Autodesk Fusion 360 part; units mm, degrees
(part 8 of 12)
  line L2696 (39.3845, 201.3731) -> (39.3845, 206.3731)
  line L2697 (39.3845, 206.3731) -> (35.0544, 208.8731)
  line L2698 (45.7146, 208.8731) -> (41.3845, 206.3731)
  line L2699 (41.3845, 206.3731) -> (41.3845, 201.3731)
  line L2700 (41.3845, 201.3731) -> (45.7146, 198.8731)
  line L2701 (45.7146, 198.8731) -> (50.0447, 201.3731)
  line L2702 (50.0447, 201.3731) -> (50.0447, 206.3731)
  line L2703 (50.0447, 206.3731) -> (45.7146, 208.8731)
  line L2704 (56.3749, 208.8731) -> (52.0447, 206.3731)
  line L2705 (52.0447, 206.3731) -> (52.0447, 201.3731)
  line L2706 (52.0447, 201.3731) -> (56.3749, 198.8731)
  line L2707 (56.3749, 198.8731) -> (60.705, 201.3731)
  line L2708 (60.705, 201.3731) -> (60.705, 206.3731)
  line L2709 (60.705, 206.3731) -> (56.3749, 208.8731)
  line L2710 (-151.5001, 218.1051) -> (-155.8302, 215.6051)
  line L2711 (-155.8302, 215.6051) -> (-155.8302, 210.6051)
  line L2712 (-155.8302, 210.6051) -> (-151.5001, 208.1051)
  line L2713 (-151.5001, 208.1051) -> (-147.17, 210.6051)
  line L2714 (-147.17, 210.6051) -> (-147.17, 215.6051)
  line L2715 (-147.17, 215.6051) -> (-151.5001, 218.1051)
  line L2716 (-140.8398, 218.1051) -> (-145.17, 215.6051)
  line L2717 (-145.17, 215.6051) -> (-145.17, 210.6051)
  line L2718 (-145.17, 210.6051) -> (-140.8398, 208.1051)
  line L2719 (-140.8398, 208.1051) -> (-136.5097, 210.6051)
  line L2720 (-136.5097, 210.6051) -> (-136.5097, 215.6051)
  line L2721 (-136.5097, 215.6051) -> (-140.8398, 218.1051)
  line L2722 (-130.1796, 218.1051) -> (-134.5097, 215.6051)
  line L2723 (-134.5097, 215.6051) -> (-134.5097, 210.6051)
  line L2724 (-134.5097, 210.6051) -> (-130.1796, 208.1051)
  line L2725 (-130.1796, 208.1051) -> (-125.8494, 210.6051)
  line L2726 (-125.8494, 210.6051) -> (-125.8494, 215.6051)
  line L2727 (-125.8494, 215.6051) -> (-130.1796, 218.1051)
  line L2728 (-119.5193, 218.1051) -> (-123.8494, 215.6051)
  line L2729 (-123.8494, 215.6051) -> (-123.8494, 210.6051)
  line L2730 (-123.8494, 210.6051) -> (-119.5193, 208.1051)
  line L2731 (-119.5193, 208.1051) -> (-115.1892, 210.6051)
  line L2732 (-115.1892, 210.6051) -> (-115.1892, 215.6051)
  line L2733 (-115.1892, 215.6051) -> (-119.5193, 218.1051)
  line L2734 (-108.8591, 218.1051) -> (-113.1892, 215.6051)
  line L2735 (-113.1892, 215.6051) -> (-113.1892, 210.6051)
  line L2736 (-113.1892, 210.6051) -> (-108.8591, 208.1051)
  line L2737 (-108.8591, 208.1051) -> (-104.5289, 210.6051)
  line L2738 (-104.5289, 210.6051) -> (-104.5289, 215.6051)
  line L2739 (-104.5289, 215.6051) -> (-108.8591, 218.1051)
  line L2740 (-98.1988, 218.1051) -> (-102.5289, 215.6051)
  line L2741 (-102.5289, 215.6051) -> (-102.5289, 210.6051)
  line L2742 (-102.5289, 210.6051) -> (-98.1988, 208.1051)
  line L2743 (-98.1988, 208.1051) -> (-93.8687, 210.6051)
  line L2744 (-93.8687, 210.6051) -> (-93.8687, 215.6051)
  line L2745 (-93.8687, 215.6051) -> (-98.1988, 218.1051)
  line L2746 (-87.5386, 218.1051) -> (-91.8687, 215.6051)
  line L2747 (-91.8687, 215.6051) -> (-91.8687, 210.6051)
  line L2748 (-91.8687, 210.6051) -> (-87.5386, 208.1051)
  line L2749 (-87.5386, 208.1051) -> (-83.2084, 210.6051)
  line L2750 (-83.2084, 210.6051) -> (-83.2084, 215.6051)
  line L2751 (-83.2084, 215.6051) -> (-87.5386, 218.1051)
  line L2752 (-76.8783, 218.1051) -> (-81.2084, 215.6051)
  line L2753 (-81.2084, 215.6051) -> (-81.2084, 210.6051)
  line L2754 (-81.2084, 210.6051) -> (-76.8783, 208.1051)
  line L2755 (-76.8783, 208.1051) -> (-72.5482, 210.6051)
  line L2756 (-72.5482, 210.6051) -> (-72.5482, 215.6051)
  line L2757 (-72.5482, 215.6051) -> (-76.8783, 218.1051)
  line L2758 (-66.218, 218.1051) -> (-70.5482, 215.6051)
  line L2759 (-70.5482, 215.6051) -> (-70.5482, 210.6051)
  line L2760 (-70.5482, 210.6051) -> (-66.218, 208.1051)
  line L2761 (-66.218, 208.1051) -> (-61.8879, 210.6051)
  line L2762 (-61.8879, 210.6051) -> (-61.8879, 215.6051)
  line L2763 (-61.8879, 215.6051) -> (-66.218, 218.1051)
  line L2764 (-55.5578, 218.1051) -> (-59.8879, 215.6051)
  line L2765 (-59.8879, 215.6051) -> (-59.8879, 210.6051)
  line L2766 (-59.8879, 210.6051) -> (-55.5578, 208.1051)
  line L2767 (-55.5578, 208.1051) -> (-51.2277, 210.6051)
  line L2768 (-51.2277, 210.6051) -> (-51.2277, 215.6051)
  line L2769 (-51.2277, 215.6051) -> (-55.5578, 218.1051)
  line L2770 (-44.8975, 218.1051) -> (-49.2277, 215.6051)
  line L2771 (-49.2277, 215.6051) -> (-49.2277, 210.6051)
  line L2772 (-49.2277, 210.6051) -> (-44.8975, 208.1051)
  line L2773 (-44.8975, 208.1051) -> (-40.5674, 210.6051)
  line L2774 (-40.5674, 210.6051) -> (-40.5674, 215.6051)
  line L2775 (-40.5674, 215.6051) -> (-44.8975, 218.1051)
  line L2776 (-34.2373, 218.1051) -> (-38.5674, 215.6051)
  line L2777 (-38.5674, 215.6051) -> (-38.5674, 210.6051)
  line L2778 (-38.5674, 210.6051) -> (-34.2373, 208.1051)
  line L2779 (-34.2373, 208.1051) -> (-29.9072, 210.6051)
  line L2780 (-29.9072, 210.6051) -> (-29.9072, 215.6051)
  line L2781 (-29.9072, 215.6051) -> (-34.2373, 218.1051)
  line L2782 (-23.577, 218.1051) -> (-27.9072, 215.6051)
  line L2783 (-27.9072, 215.6051) -> (-27.9072, 210.6051)
  line L2784 (-27.9072, 210.6051) -> (-23.577, 208.1051)
  line L2785 (-23.577, 208.1051) -> (-19.2469, 210.6051)
  line L2786 (-19.2469, 210.6051) -> (-19.2469, 215.6051)
  line L2787 (-19.2469, 215.6051) -> (-23.577, 218.1051)
  line L2788 (-12.9168, 218.1051) -> (-17.2469, 215.6051)
  line L2789 (-17.2469, 215.6051) -> (-17.2469, 210.6051)
  line L2790 (-17.2469, 210.6051) -> (-12.9168, 208.1051)
  line L2791 (-12.9168, 208.1051) -> (-8.5866, 210.6051)
  line L2792 (-8.5866, 210.6051) -> (-8.5866, 215.6051)
  line L2793 (-8.5866, 215.6051) -> (-12.9168, 218.1051)
  line L2794 (-2.2565, 218.1051) -> (-6.5866, 215.6051)
  line L2795 (-6.5866, 215.6051) -> (-6.5866, 210.6051)
  line L2796 (-6.5866, 210.6051) -> (-2.2565, 208.1051)
  line L2797 (-2.2565, 208.1051) -> (2.0736, 210.6051)
  line L2798 (2.0736, 210.6051) -> (2.0736, 215.6051)
  line L2799 (2.0736, 215.6051) -> (-2.2565, 218.1051)
  line L2800 (8.4037, 218.1051) -> (4.0736, 215.6051)
  line L2801 (4.0736, 215.6051) -> (4.0736, 210.6051)
  line L2802 (4.0736, 210.6051) -> (8.4037, 208.1051)
  line L2803 (8.4037, 208.1051) -> (12.7339, 210.6051)
  line L2804 (12.7339, 210.6051) -> (12.7339, 215.6051)
  line L2805 (12.7339, 215.6051) -> (8.4037, 218.1051)
  line L2806 (19.064, 218.1051) -> (14.7339, 215.6051)
  line L2807 (14.7339, 215.6051) -> (14.7339, 210.6051)
  line L2808 (14.7339, 210.6051) -> (19.064, 208.1051)
  line L2809 (19.064, 208.1051) -> (23.3941, 210.6051)
  line L2810 (23.3941, 210.6051) -> (23.3941, 215.6051)
  line L2811 (23.3941, 215.6051) -> (19.064, 218.1051)
  line L2812 (29.7242, 218.1051) -> (25.3941, 215.6051)
  line L2813 (25.3941, 215.6051) -> (25.3941, 210.6051)
  line L2814 (25.3941, 210.6051) -> (29.7242, 208.1051)
  line L2815 (29.7242, 208.1051) -> (34.0544, 210.6051)
  line L2816 (34.0544, 210.6051) -> (34.0544, 215.6051)
  line L2817 (34.0544, 215.6051) -> (29.7242, 218.1051)
  line L2818 (40.3845, 218.1051) -> (36.0544, 215.6051)
  line L2819 (36.0544, 215.6051) -> (36.0544, 210.6051)
  line L2820 (36.0544, 210.6051) -> (40.3845, 208.1051)
  line L2821 (40.3845, 208.1051) -> (44.7146, 210.6051)
  line L2822 (44.7146, 210.6051) -> (44.7146, 215.6051)
  line L2823 (44.7146, 215.6051) -> (40.3845, 218.1051)
  line L2824 (51.0447, 218.1051) -> (46.7146, 215.6051)
  line L2825 (46.7146, 215.6051) -> (46.7146, 210.6051)
  line L2826 (46.7146, 210.6051) -> (51.0447, 208.1051)
  line L2827 (51.0447, 208.1051) -> (55.3749, 210.6051)
  line L2828 (55.3749, 210.6051) -> (55.3749, 215.6051)
  line L2829 (55.3749, 215.6051) -> (51.0447, 218.1051)
  line L2830 (61.705, 218.1051) -> (57.3749, 215.6051)
  line L2831 (57.3749, 215.6051) -> (57.3749, 210.6051)
  line L2832 (57.3749, 210.6051) -> (61.705, 208.1051)
  line L2833 (61.705, 208.1051) -> (66.0351, 210.6051)
  line L2834 (66.0351, 210.6051) -> (66.0351, 215.6051)
  line L2835 (66.0351, 215.6051) -> (61.705, 218.1051)
  line L2836 (-146.17, 227.3372) -> (-150.5001, 224.8372)
  line L2837 (-150.5001, 224.8372) -> (-150.5001, 219.8372)
  line L2838 (-150.5001, 219.8372) -> (-146.17, 217.3372)
  line L2839 (-146.17, 217.3372) -> (-141.8398, 219.8372)
  line L2840 (-141.8398, 219.8372) -> (-141.8398, 224.8372)
  line L2841 (-141.8398, 224.8372) -> (-146.17, 227.3372)
  line L2842 (-135.5097, 227.3372) -> (-139.8398, 224.8372)
  line L2843 (-139.8398, 224.8372) -> (-139.8398, 219.8372)
  line L2844 (-139.8398, 219.8372) -> (-135.5097, 217.3372)
  line L2845 (-135.5097, 217.3372) -> (-131.1796, 219.8372)
  line L2846 (-131.1796, 219.8372) -> (-131.1796, 224.8372)
  line L2847 (-131.1796, 224.8372) -> (-135.5097, 227.3372)
  line L2848 (-124.8494, 227.3372) -> (-129.1796, 224.8372)
  line L2849 (-129.1796, 224.8372) -> (-129.1796, 219.8372)
  line L2850 (-129.1796, 219.8372) -> (-124.8494, 217.3372)
  line L2851 (-124.8494, 217.3372) -> (-120.5193, 219.8372)
  line L2852 (-120.5193, 219.8372) -> (-120.5193, 224.8372)
  line L2853 (-120.5193, 224.8372) -> (-124.8494, 227.3372)
  line L2854 (-114.1892, 227.3372) -> (-118.5193, 224.8372)
  line L2855 (-118.5193, 224.8372) -> (-118.5193, 219.8372)
  line L2856 (-118.5193, 219.8372) -> (-114.1892, 217.3372)
  line L2857 (-114.1892, 217.3372) -> (-109.8591, 219.8372)
  line L2858 (-109.8591, 219.8372) -> (-109.8591, 224.8372)
  line L2859 (-109.8591, 224.8372) -> (-114.1892, 227.3372)
  line L2860 (-103.5289, 227.3372) -> (-107.8591, 224.8372)
  line L2861 (-107.8591, 224.8372) -> (-107.8591, 219.8372)
  line L2862 (-107.8591, 219.8372) -> (-103.5289, 217.3372)
  line L2863 (-103.5289, 217.3372) -> (-99.1988, 219.8372)
  line L2864 (-99.1988, 219.8372) -> (-99.1988, 224.8372)
  line L2865 (-99.1988, 224.8372) -> (-103.5289, 227.3372)
  line L2866 (-92.8687, 227.3372) -> (-97.1988, 224.8372)
  line L2867 (-97.1988, 224.8372) -> (-97.1988, 219.8372)
  line L2868 (-97.1988, 219.8372) -> (-92.8687, 217.3372)
  line L2869 (-92.8687, 217.3372) -> (-88.5386, 219.8372)
  line L2870 (-88.5386, 219.8372) -> (-88.5386, 224.8372)
  line L2871 (-88.5386, 224.8372) -> (-92.8687, 227.3372)
  line L2872 (-82.2084, 227.3372) -> (-86.5386, 224.8372)
  line L2873 (-86.5386, 224.8372) -> (-86.5386, 219.8372)
  line L2874 (-86.5386, 219.8372) -> (-82.2084, 217.3372)
  line L2875 (-82.2084, 217.3372) -> (-77.8783, 219.8372)
  line L2876 (-77.8783, 219.8372) -> (-77.8783, 224.8372)
  line L2877 (-77.8783, 224.8372) -> (-82.2084, 227.3372)
  line L2878 (-71.5482, 227.3372) -> (-75.8783, 224.8372)
  line L2879 (-75.8783, 224.8372) -> (-75.8783, 219.8372)
  line L2880 (-75.8783, 219.8372) -> (-71.5482, 217.3372)
  line L2881 (-71.5482, 217.3372) -> (-67.218, 219.8372)
  line L2882 (-67.218, 219.8372) -> (-67.218, 224.8372)
  line L2883 (-67.218, 224.8372) -> (-71.5482, 227.3372)
  line L2884 (-60.8879, 227.3372) -> (-65.218, 224.8372)
  line L2885 (-65.218, 224.8372) -> (-65.218, 219.8372)
  line L2886 (-65.218, 219.8372) -> (-60.8879, 217.3372)
  line L2887 (-60.8879, 217.3372) -> (-56.5578, 219.8372)
  line L2888 (-56.5578, 219.8372) -> (-56.5578, 224.8372)
  line L2889 (-56.5578, 224.8372) -> (-60.8879, 227.3372)
  line L2890 (-50.2277, 227.3372) -> (-54.5578, 224.8372)
  line L2891 (-54.5578, 224.8372) -> (-54.5578, 219.8372)
  line L2892 (-54.5578, 219.8372) -> (-50.2277, 217.3372)
  line L2893 (-50.2277, 217.3372) -> (-45.8975, 219.8372)
  line L2894 (-45.8975, 219.8372) -> (-45.8975, 224.8372)
  line L2895 (-45.8975, 224.8372) -> (-50.2277, 227.3372)
  line L2896 (-39.5674, 227.3372) -> (-43.8975, 224.8372)
  line L2897 (-43.8975, 224.8372) -> (-43.8975, 219.8372)
  line L2898 (-43.8975, 219.8372) -> (-39.5674, 217.3372)
  line L2899 (-39.5674, 217.3372) -> (-35.2373, 219.8372)
  line L2900 (-35.2373, 219.8372) -> (-35.2373, 224.8372)
  line L2901 (-35.2373, 224.8372) -> (-39.5674, 227.3372)
  line L2902 (-28.9072, 227.3372) -> (-33.2373, 224.8372)
  line L2903 (-33.2373, 224.8372) -> (-33.2373, 219.8372)
  line L2904 (-33.2373, 219.8372) -> (-28.9072, 217.3372)
  line L2905 (-28.9072, 217.3372) -> (-24.577, 219.8372)
  line L2906 (-24.577, 219.8372) -> (-24.577, 224.8372)
  line L2907 (-24.577, 224.8372) -> (-28.9072, 227.3372)
  line L2908 (-18.2469, 227.3372) -> (-22.577, 224.8372)
  line L2909 (-22.577, 224.8372) -> (-22.577, 219.8372)
  line L2910 (-22.577, 219.8372) -> (-18.2469, 217.3372)
  line L2911 (-18.2469, 217.3372) -> (-13.9168, 219.8372)
  line L2912 (-13.9168, 219.8372) -> (-13.9168, 224.8372)
  line L2913 (-13.9168, 224.8372) -> (-18.2469, 227.3372)
  line L2914 (-7.5866, 227.3372) -> (-11.9168, 224.8372)
  line L2915 (-11.9168, 224.8372) -> (-11.9168, 219.8372)
  line L2916 (-11.9168, 219.8372) -> (-7.5866, 217.3372)
  line L2917 (-7.5866, 217.3372) -> (-3.2565, 219.8372)
  line L2918 (-3.2565, 219.8372) -> (-3.2565, 224.8372)
  line L2919 (-3.2565, 224.8372) -> (-7.5866, 227.3372)
  line L2920 (3.0736, 227.3372) -> (-1.2565, 224.8372)
  line L2921 (-1.2565, 224.8372) -> (-1.2565, 219.8372)
  line L2922 (-1.2565, 219.8372) -> (3.0736, 217.3372)
  line L2923 (3.0736, 217.3372) -> (7.4037, 219.8372)
  line L2924 (7.4037, 219.8372) -> (7.4037, 224.8372)
  line L2925 (7.4037, 224.8372) -> (3.0736, 227.3372)
  line L2926 (13.7339, 227.3372) -> (9.4037, 224.8372)
  line L2927 (9.4037, 224.8372) -> (9.4037, 219.8372)
  line L2928 (9.4037, 219.8372) -> (13.7339, 217.3372)
  line L2929 (13.7339, 217.3372) -> (18.064, 219.8372)
  line L2930 (18.064, 219.8372) -> (18.064, 224.8372)
  line L2931 (18.064, 224.8372) -> (13.7339, 227.3372)
  line L2932 (24.3941, 227.3372) -> (20.064, 224.8372)
  line L2933 (20.064, 224.8372) -> (20.064, 219.8372)
  line L2934 (20.064, 219.8372) -> (24.3941, 217.3372)
  line L2935 (24.3941, 217.3372) -> (28.7242, 219.8372)
  line L2936 (28.7242, 219.8372) -> (28.7242, 224.8372)
  line L2937 (28.7242, 224.8372) -> (24.3941, 227.3372)
  line L2938 (35.0544, 227.3372) -> (30.7242, 224.8372)
  line L2939 (30.7242, 224.8372) -> (30.7242, 219.8372)
  line L2940 (30.7242, 219.8372) -> (35.0544, 217.3372)
  line L2941 (35.0544, 217.3372) -> (39.3845, 219.8372)
  line L2942 (39.3845, 219.8372) -> (39.3845, 224.8372)
  line L2943 (39.3845, 224.8372) -> (35.0544, 227.3372)
  line L2944 (45.7146, 227.3372) -> (41.3845, 224.8372)
  line L2945 (41.3845, 224.8372) -> (41.3845, 219.8372)
  line L2946 (41.3845, 219.8372) -> (45.7146, 217.3372)
  line L2947 (45.7146, 217.3372) -> (50.0447, 219.8372)
  line L2948 (50.0447, 219.8372) -> (50.0447, 224.8372)
  line L2949 (50.0447, 224.8372) -> (45.7146, 227.3372)
  line L2950 (56.3749, 227.3372) -> (52.0447, 224.8372)
  line L2951 (52.0447, 224.8372) -> (52.0447, 219.8372)
  line L2952 (52.0447, 219.8372) -> (56.3749, 217.3372)
  line L2953 (56.3749, 217.3372) -> (60.705, 219.8372)
  line L2954 (60.705, 219.8372) -> (60.705, 224.8372)
  line L2955 (60.705, 224.8372) -> (56.3749, 227.3372)
  line L2956 (-151.5001, 236.5692) -> (-155.8302, 234.0692)
  line L2957 (-155.8302, 234.0692) -> (-155.8302, 229.0692)
  line L2958 (-155.8302, 229.0692) -> (-151.5001, 226.5692)
  line L2959 (-151.5001, 226.5692) -> (-147.17, 229.0692)
  line L2960 (-147.17, 229.0692) -> (-147.17, 234.0692)
  line L2961 (-147.17, 234.0692) -> (-151.5001, 236.5692)
  line L2962 (-140.8398, 236.5692) -> (-145.17, 234.0692)
  line L2963 (-145.17, 234.0692) -> (-145.17, 229.0692)
  line L2964 (-145.17, 229.0692) -> (-140.8398, 226.5692)
  line L2965 (-140.8398, 226.5692) -> (-136.5097, 229.0692)
  line L2966 (-136.5097, 229.0692) -> (-136.5097, 234.0692)
  line L2967 (-136.5097, 234.0692) -> (-140.8398, 236.5692)
  line L2968 (-130.1796, 236.5692) -> (-134.5097, 234.0692)
  line L2969 (-134.5097, 234.0692) -> (-134.5097, 229.0692)
  line L2970 (-134.5097, 229.0692) -> (-130.1796, 226.5692)
  line L2971 (-130.1796, 226.5692) -> (-125.8494, 229.0692)
  line L2972 (-125.8494, 229.0692) -> (-125.8494, 234.0692)
  line L2973 (-125.8494, 234.0692) -> (-130.1796, 236.5692)
  line L2974 (-119.5193, 236.5692) -> (-123.8494, 234.0692)
  line L2975 (-123.8494, 234.0692) -> (-123.8494, 229.0692)
  line L2976 (-123.8494, 229.0692) -> (-119.5193, 226.5692)
  line L2977 (-119.5193, 226.5692) -> (-115.1892, 229.0692)
  line L2978 (-115.1892, 229.0692) -> (-115.1892, 234.0692)
  line L2979 (-115.1892, 234.0692) -> (-119.5193, 236.5692)
  line L2980 (-108.8591, 236.5692) -> (-113.1892, 234.0692)
  line L2981 (-113.1892, 234.0692) -> (-113.1892, 229.0692)
  line L2982 (-113.1892, 229.0692) -> (-108.8591, 226.5692)
  line L2983 (-108.8591, 226.5692) -> (-104.5289, 229.0692)
  line L2984 (-104.5289, 229.0692) -> (-104.5289, 234.0692)
  line L2985 (-104.5289, 234.0692) -> (-108.8591, 236.5692)
  line L2986 (-98.1988, 236.5692) -> (-102.5289, 234.0692)
  line L2987 (-102.5289, 234.0692) -> (-102.5289, 229.0692)
  line L2988 (-102.5289, 229.0692) -> (-98.1988, 226.5692)
  line L2989 (-98.1988, 226.5692) -> (-93.8687, 229.0692)
  line L2990 (-93.8687, 229.0692) -> (-93.8687, 234.0692)
  line L2991 (-93.8687, 234.0692) -> (-98.1988, 236.5692)
  line L2992 (-87.5386, 236.5692) -> (-91.8687, 234.0692)
  line L2993 (-91.8687, 234.0692) -> (-91.8687, 229.0692)
  line L2994 (-91.8687, 229.0692) -> (-87.5386, 226.5692)
  line L2995 (-87.5386, 226.5692) -> (-83.2084, 229.0692)
  line L2996 (-83.2084, 229.0692) -> (-83.2084, 234.0692)
  line L2997 (-83.2084, 234.0692) -> (-87.5386, 236.5692)
  line L2998 (-76.8783, 236.5692) -> (-81.2084, 234.0692)
  line L2999 (-81.2084, 234.0692) -> (-81.2084, 229.0692)
  line L3000 (-81.2084, 229.0692) -> (-76.8783, 226.5692)
  line L3001 (-76.8783, 226.5692) -> (-72.5482, 229.0692)
  line L3002 (-72.5482, 229.0692) -> (-72.5482, 234.0692)
  line L3003 (-72.5482, 234.0692) -> (-76.8783, 236.5692)
  line L3004 (-66.218, 236.5692) -> (-70.5482, 234.0692)
  line L3005 (-70.5482, 234.0692) -> (-70.5482, 229.0692)
  line L3006 (-70.5482, 229.0692) -> (-66.218, 226.5692)
  line L3007 (-66.218, 226.5692) -> (-61.8879, 229.0692)
  line L3008 (-61.8879, 229.0692) -> (-61.8879, 234.0692)
  line L3009 (-61.8879, 234.0692) -> (-66.218, 236.5692)
  line L3010 (-55.5578, 236.5692) -> (-59.8879, 234.0692)
  line L3011 (-59.8879, 234.0692) -> (-59.8879, 229.0692)
  line L3012 (-59.8879, 229.0692) -> (-55.5578, 226.5692)
  line L3013 (-55.5578, 226.5692) -> (-51.2277, 229.0692)
  line L3014 (-51.2277, 229.0692) -> (-51.2277, 234.0692)
  line L3015 (-51.2277, 234.0692) -> (-55.5578, 236.5692)
  line L3016 (-44.8975, 236.5692) -> (-49.2277, 234.0692)
  line L3017 (-49.2277, 234.0692) -> (-49.2277, 229.0692)
  line L3018 (-49.2277, 229.0692) -> (-44.8975, 226.5692)
  line L3019 (-44.8975, 226.5692) -> (-40.5674, 229.0692)
  line L3020 (-40.5674, 229.0692) -> (-40.5674, 234.0692)
  line L3021 (-40.5674, 234.0692) -> (-44.8975, 236.5692)
  line L3022 (-34.2373, 236.5692) -> (-38.5674, 234.0692)
  line L3023 (-38.5674, 234.0692) -> (-38.5674, 229.0692)
  line L3024 (-38.5674, 229.0692) -> (-34.2373, 226.5692)
  line L3025 (-34.2373, 226.5692) -> (-29.9072, 229.0692)
  line L3026 (-29.9072, 229.0692) -> (-29.9072, 234.0692)
  line L3027 (-29.9072, 234.0692) -> (-34.2373, 236.5692)
  line L3028 (-23.577, 236.5692) -> (-27.9072, 234.0692)
  line L3029 (-27.9072, 234.0692) -> (-27.9072, 229.0692)
  line L3030 (-27.9072, 229.0692) -> (-23.577, 226.5692)
  line L3031 (-23.577, 226.5692) -> (-19.2469, 229.0692)
  line L3032 (-19.2469, 229.0692) -> (-19.2469, 234.0692)
  line L3033 (-19.2469, 234.0692) -> (-23.577, 236.5692)
  line L3034 (-12.9168, 236.5692) -> (-17.2469, 234.0692)
  line L3035 (-17.2469, 234.0692) -> (-17.2469, 229.0692)
  line L3036 (-17.2469, 229.0692) -> (-12.9168, 226.5692)
  line L3037 (-12.9168, 226.5692) -> (-8.5866, 229.0692)
  line L3038 (-8.5866, 229.0692) -> (-8.5866, 234.0692)
  line L3039 (-8.5866, 234.0692) -> (-12.9168, 236.5692)
  line L3040 (-2.2565, 236.5692) -> (-6.5866, 234.0692)
  line L3041 (-6.5866, 234.0692) -> (-6.5866, 229.0692)
  line L3042 (-6.5866, 229.0692) -> (-2.2565, 226.5692)
  line L3043 (-2.2565, 226.5692) -> (2.0736, 229.0692)
  line L3044 (2.0736, 229.0692) -> (2.0736, 234.0692)
  line L3045 (2.0736, 234.0692) -> (-2.2565, 236.5692)
  line L3046 (8.4037, 236.5692) -> (4.0736, 234.0692)
  line L3047 (4.0736, 234.0692) -> (4.0736, 229.0692)
  line L3048 (4.0736, 229.0692) -> (8.4037, 226.5692)
  line L3049 (8.4037, 226.5692) -> (12.7339, 229.0692)
  line L3050 (12.7339, 229.0692) -> (12.7339, 234.0692)
  line L3051 (12.7339, 234.0692) -> (8.4037, 236.5692)
  line L3052 (19.064, 236.5692) -> (14.7339, 234.0692)
  line L3053 (14.7339, 234.0692) -> (14.7339, 229.0692)
  line L3054 (14.7339, 229.0692) -> (19.064, 226.5692)
  line L3055 (19.064, 226.5692) -> (23.3941, 229.0692)
  line L3056 (23.3941, 229.0692) -> (23.3941, 234.0692)
  line L3057 (23.3941, 234.0692) -> (19.064, 236.5692)
  line L3058 (29.7242, 236.5692) -> (25.3941, 234.0692)
  line L3059 (25.3941, 234.0692) -> (25.3941, 229.0692)
  line L3060 (25.3941, 229.0692) -> (29.7242, 226.5692)
  line L3061 (29.7242, 226.5692) -> (34.0544, 229.0692)
  line L3062 (34.0544, 229.0692) -> (34.0544, 234.0692)
  line L3063 (34.0544, 234.0692) -> (29.7242, 236.5692)
  line L3064 (40.3845, 236.5692) -> (36.0544, 234.0692)
  line L3065 (36.0544, 234.0692) -> (36.0544, 229.0692)
  line L3066 (36.0544, 229.0692) -> (40.3845, 226.5692)
  line L3067 (40.3845, 226.5692) -> (44.7146, 229.0692)
  line L3068 (44.7146, 229.0692) -> (44.7146, 234.0692)
  line L3069 (44.7146, 234.0692) -> (40.3845, 236.5692)
  line L3070 (51.0447, 236.5692) -> (46.7146, 234.0692)
  line L3071 (46.7146, 234.0692) -> (46.7146, 229.0692)
  line L3072 (46.7146, 229.0692) -> (51.0447, 226.5692)
  line L3073 (51.0447, 226.5692) -> (55.3749, 229.0692)
  line L3074 (55.3749, 229.0692) -> (55.3749, 234.0692)
  line L3075 (55.3749, 234.0692) -> (51.0447, 236.5692)
  line L3076 (61.705, 236.5692) -> (57.3749, 234.0692)
  line L3077 (57.3749, 234.0692) -> (57.3749, 229.0692)
  line L3078 (57.3749, 229.0692) -> (61.705, 226.5692)
  line L3079 (61.705, 226.5692) -> (66.0351, 229.0692)
  line L3080 (66.0351, 229.0692) -> (66.0351, 234.0692)
  line L3081 (66.0351, 234.0692) -> (61.705, 236.5692)
extrude "拉伸6" cut sketch "草图29" against normal blind 4 contours L4 L5 L6 L7 L8 L9 | L10 L11 L12 L13 L14 L15 | L16 L17 L18 L19 L20 L21 | L22 L23 L24 L25 L26 L27 | L28 L29 L30 L31 L32 L33 | L34 L35 L36 L37 L38 L39 | L40 L41 L42 L43 L44 L45 | L46 L47 L48 L49 L50 L51 | L52 L53 L54 L55 L56 L57 | L58 L59 L60 L61 L62 L63 | L64 L65 L66 L67 L68 L69 | L70 L71 L72 L73 L74 L75 | L76 L77 L78 L79 L80 L81 | L82 L83 L84 L85 L86 L87 | L88 L89 L90 L91 L92 L93 | L94 L95 L96 L97 L98 L99 | L100 L101 L102 L103 L104 L105 | L106 L107 L108 L109 L110 L111 | L112 L113 L114 L115 L116 L117 | L118 L119 L120 L121 L122 L123 | L124 L125 L126 L127 L128 L129 | L130 L131 L132 L133 L134 L135 | L136 L137 L138 L139 L140 L141 | L142 L143 L144 L145 L146 L147 | L148 L149 L150 L151 L152 L153 | L154 L155 L156 L157 L158 L159 | L160 L161 L162 L163 L164 L165 | L166 L167 L168 L169 L170 L171 | L172 L173 L174 L175 L176 L177 | L178 L179 L180 L181 L182 L183 | L184 L185 L186 L187 L188 L189 | L190 L191 L192 L193 L194 L195 | L196 L197 L198 L199 L200 L201 | L202 L203 L204 L205 L206 L207 | L208 L209 L210 L211 L212 L213 | L214 L215 L216 L217 L218 L219 | L220 L221 L222 L223 L224 L225 | L226 L227 L228 L229 L230 L231 | L232 L233 L234 L235 L236 L237 | L238 L239 L240 L241 L242 L243 | L244 L245 L246 L247 L248 L249 | L250 L251 L252 L253 L254 L255 | L256 L257 L258 L259 L260 L261 | L262 L263 L264 L265 L266 L267 | L268 L269 L270 L271 L272 L273 | L274 L275 L276 L277 L278 L279 | L280 L281 L282 L283 L284 L285 | L286 L287 L288 L289 L290 L291 | L292 L293 L294 L295 L296 L297 | L298 L299 L300 L301 L302 L303 | L304 L305 L306 L307 L308 L309 | L310 L311 L312 L313 L314 L315 | L316 L317 L318 L319 L320 L321 | L322 L323 L324 L325 L326 L327 | L328 L329 L330 L331 L332 L333 | L334 L335 L336 L337 L338 L339 | L340 L341 L342 L343 L344 L345 | L346 L347 L348 L349 L350 L351 | L352 L353 L354 L355 L356 L357 | L358 L359 L360 L361 L362 L363 | L364 L365 L366 L367 L368 L369 | L370 L371 L372 L373 L374 L375 | L376 L377 L378 L379 L380 L381 | L382 L383 L384 L385 L386 L387 | L388 L389 L390 L391 L392 L393 | L394 L395 L396 L397 L398 L399 | L400 L401 L402 L403 L404 L405 | L406 L407 L408 L409 L410 L411 | L412 L413 L414 L415 L416 L417 | L418 L419 L420 L421 L422 L423 | L424 L425 L426 L427 L428 L429 | L430 L431 L432 L433 L434 L435 | L436 L437 L438 L439 L440 L441 | L442 L443 L444 L445 L446 L447 | L448 L449 L450 L451 L452 L453 | L454 L455 L456 L457 L458 L459 | L460 L461 L462 L463 L464 L465 | L466 L467 L468 L469 L470 L471 | L472 L473 L474 L475 L476 L477 | L478 L479 L480 L481 L482 L483 | L484 L485 L486 L487 L488 L489 | L490 L491 L492 L493 L494 L495 | L496 L497 L498 L499 L500 L501 | L502 L503 L504 L505 L506 L507 | L508 L509 L510 L511 L512 L513 | L514 L515 L516 L517 L518 L519 | L520 L521 L522 L523 L524 L525 | L526 L527 L528 L529 L530 L531 | L532 L533 L534 L535 L536 L537 | L538 L539 L540 L541 L542 L543 | L544 L545 L546 L547 L548 L549 | L550 L551 L552 L553 L554 L555 | L556 L557 L558 L559 L560 L561 | L562 L563 L564 L565 L566 L567 | L568 L569 L570 L571 L572 L573 | L574 L575 L576 L577 L578 L579 | L580 L581 L582 L583 L584 L585 | L586 L587 L588 L589 L590 L591 | L592 L593 L594 L595 L596 L597 | L598 L599 L600 L601 L602 L603 | L604 L605 L606 L607 L608 L609 | L610 L611 L612 L613 L614 L615 | L616 L617 L618 L619 L620 L621 | L622 L623 L624 L625 L626 L627 | L628 L629 L630 L631 L632 L633 | L634 L635 L636 L637 L638 L639 | L640 L641 L642 L643 L644 L645 | L646 L647 L648 L649 L650 L651 | L652 L653 L654 L655 L656 L657 | L658 L659 L660 L661 L662 L663 | L664 L665 L666 L667 L668 L669 | L670 L671 L672 L673 L674 L675 | L676 L677 L678 L679 L680 L681 | L682 L683 L684 L685 L686 L687 | L688 L689 L690 L691 L692 L693 | L694 L695 L696 L697 L698 L699 | L700 L701 L702 L703 L704 L705 | L706 L707 L708 L709 L710 L711 | L712 L713 L714 L715 L716 L717 | L718 L719 L720 L721 L722 L723 | L724 L725 L726 L727 L728 L729 | L730 L731 L732 L733 L734 L735 | L736 L737 L738 L739 L740 L741 | L742 L743 L744 L745 L746 L747 | L748 L749 L750 L751 L752 L753 | L754 L755 L756 L757 L758 L759 | L760 L761 L762 L763 L764 L765 | L766 L767 L768 L769 L770 L771 | L772 L773 L774 L775 L776 L777 | L778 L779 L780 L781 L782 L783 | L784 L785 L786 L787 L788 L789 | L790 L791 L792 L793 L794 L795 | L796 L797 L798 L799 L800 L801 | L802 L803 L804 L805 L806 L807 | L808 L809 L810 L811 L812 L813 | L814 L815 L816 L817 L818 L819 | L820 L821 L822 L823 L824 L825 | L826 L827 L828 L829 L830 L831 | L832 L833 L834 L835 L836 L837 | L838 L839 L840 L841 L842 L843 | L844 L845 L846 L847 L848 L849 | L850 L851 L852 L853 L854 L855 | L856 L857 L858 L859 L860 L861 | L862 L863 L864 L865 L866 L867 | L868 L869 L870 L871 L872 L873 | L874 L875 L876 L877 L878 L879 | L880 L881 L882 L883 L884 L885 | L886 L887 L888 L889 L890 L891 | L892 L893 L894 L895 L896 L897 | L898 L899 L900 L901 L902 L903 | L904 L905 L906 L907 L908 L909 | L910 L911 L912 L913 L914 L915 | L916 L917 L918 L919 L920 L921 | L922 L923 L924 L925 L926 L927 | L928 L929 L930 L931 L932 L933 | L934 L935 L936 L937 L938 L939 | L940 L941 L942 L943 L944 L945 | L946 L947 L948 L949 L950 L951 | L952 L953 L954 L955 L956 L957 | L958 L959 L960 L961 L962 L963 | L964 L965 L966 L967 L968 L969 | L970 L971 L972 L973 L974 L975 | L976 L977 L978 L979 L980 L981 | L982 L983 L984 L985 L986 L987 | L988 L989 L990 L991 L992 L993 | L994 L995 L996 L997 L998 L999 | L1000 L1001 L1002 L1003 L1004 L1005 | L1006 L1007 L1008 L1009 L1010 L1011 | L1012 L1013 L1014 L1015 L1016 L1017 | L1018 L1019 L1020 L1021 L1022 L1023 | L1024 L1025 L1026 L1027 L1028 L1029 | L1030 L1031 L1032 L1033 L1034 L1035 | L1036 L1037 L1038 L1039 L1040 L1041 | L1042 L1043 L1044 L1045 L1046 L1047 | L1048 L1049 L1050 L1051 L1052 L1053 | L1054 L1055 L1056 L1057 L1058 L1059 | L1060 L1061 L1062 L1063 L1064 L1065 | L1066 L1067 L1068 L1069 L1070 L1071 | L1072 L1073 L1074 L1075 L1076 L1077 | L1078 L1079 L1080 L1081 L1082 L1083 | L1084 L1085 L1086 L1087 L1088 L1089 | L1090 L1091 L1092 L1093 L1094 L1095 | L1096 L1097 L1098 L1099 L1100 L1101 | L1102 L1103 L1104 L1105 L1106 L1107 | L1108 L1109 L1110 L1111 L1112 L1113 | L1114 L1115 L1116 L1117 L1118 L1119 | L1120 L1121 L1122 L1123 L1124 L1125 | L1126 L1127 L1128 L1129 L1130 L1131 | L1132 L1133 L1134 L1135 L1136 L1137 | L1138 L1139 L1140 L1141 L1142 L1143 | L1144 L1145 L1146 L1147 L1148 L1149 | L1150 L1151 L1152 L1153 L1154 L1155 | L1156 L1157 L1158 L1159 L1160 L1161 | L1162 L1163 L1164 L1165 L1166 L1167 | L1168 L1169 L1170 L1171 L1172 L1173 | L1174 L1175 L1176 L1177 L1178 L1179 | L1180 L1181 L1182 L1183 L1184 L1185 | L1186 L1187 L1188 L1189 L1190 L1191 | L1192 L1193 L1194 L1195 L1196 L1197 | L1198 L1199 L1200 L1201 L1202 L1203 | L1204 L1205 L1206 L1207 L1208 L1209 | L1210 L1211 L1212 L1213 L1214 L1215 | L1216 L1217 L1218 L1219 L1220 L1221 | L1222 L1223 L1224 L1225 L1226 L1227 | L1228 L1229 L1230 L1231 L1232 L1233 | L1234 L1235 L1236 L1237 L1238 L1239 | L1240 L1241 L1242 L1243 L1244 L1245 | L1246 L1247 L1248 L1249 L1250 L1251 | L1252 L1253 L1254 L1255 L1256 L1257 | L1258 L1259 L1260 L1261 L1262 L1263 | L1264 L1265 L1266 L1267 L1268 L1269 | L1270 L1271 L1272 L1273 L1274 L1275 | L1276 L1277 L1278 L1279 L1280 L1281 | L1282 L1283 L1284 L1285 L1286 L1287 | L1288 L1289 L1290 L1291 L1292 L1293 | L1294 L1295 L1296 L1297 L1298 L1299 | L1300 L1301 L1302 L1303 L1304 L1305 | L1306 L1307 L1308 L1309 L1310 L1311 | L1312 L1313 L1314 L1315 L1316 L1317 | L1318 L1319 L1320 L1321 L1322 L1323 | L1324 L1325 L1326 L1327 L1328 L1329 | L1330 L1331 L1332 L1333 L1334 L1335 | L1336 L1337 L1338 L1339 L1340 L1341 | L1342 L1343 L1344 L1345 L1346 L1347 | L1348 L1349 L1350 L1351 L1352 L1353 | L1354 L1355 L1356 L1357 L1358 L1359 | L1360 L1361 L1362 L1363 L1364 L1365 | L1366 L1367 L1368 L1369 L1370 L1371 | L1372 L1373 L1374 L1375 L1376 L1377 | L1378 L1379 L1380 L1381 L1382 L1383 | L1384 L1385 L1386 L1387 L1388 L1389 | L1390 L1391 L1392 L1393 L1394 L1395 | L1396 L1397 L1398 L1399 L1400 L1401 | L1402 L1403 L1404 L1405 L1406 L1407 | L1408 L1409 L1410 L1411 L1412 L1413 | L1414 L1415 L1416 L1417 L1418 L1419 | L1420 L1421 L1422 L1423 L1424 L1425 | L1426 L1427 L1428 L1429 L1430 L1431 | L1432 L1433 L1434 L1435 L1436 L1437 | L1438 L1439 L1440 L1441 L1442 L1443 | L1444 L1445 L1446 L1447 L1448 L1449 | L1450 L1451 L1452 L1453 L1454 L1455 | L1456 L1457 L1458 L1459 L1460 L1461 | L1462 L1463 L1464 L1465 L1466 L1467 | L1468 L1469 L1470 L1471 L1472 L1473 | L1474 L1475 L1476 L1477 L1478 L1479 | L1480 L1481 L1482 L1483 L1484 L1485 | L1486 L1487 L1488 L1489 L1490 L1491 | L1492 L1493 L1494 L1495 L1496 L1497 | L1498 L1499 L1500 L1501 L1502 L1503 | L1504 L1505 L1506 L1507 L1508 L1509 | L1510 L1511 L1512 L1513 L1514 L1515 | L1516 L1517 L1518 L1519 L1520 L1521 | L1522 L1523 L1524 L1525 L1526 L1527 | L1528 L1529 L1530 L1531 L1532 L1533 | L1534 L1535 L1536 L1537 L1538 L1539 | L1540 L1541 L1542 L1543 L1544 L1545 | L1546 L1547 L1548 L1549 L1550 L1551 | L1552 L1553 L1554 L1555 L1556 L1557 | L1558 L1559 L1560 L1561 L1562 L1563 | L1564 L1565 L1566 L1567 L1568 L1569 | L1570 L1571 L1572 L1573 L1574 L1575 | L1576 L1577 L1578 L1579 L1580 L1581 | L1582 L1583 L1584 L1585 L1586 L1587 | L1588 L1589 L1590 L1591 L1592 L1593 | L1594 L1595 L1596 L1597 L1598 L1599 | L1600 L1601 L1602 L1603 L1604 L1605 | L1606 L1607 L1608 L1609 L1610 L1611 | L1612 L1613 L1614 L1615 L1616 L1617 | L1618 L1619 L1620 L1621 L1622 L1623 | L1624 L1625 L1626 L1627 L1628 L1629 | L1630 L1631 L1632 L1633 L1634 L1635 | L1636 L1637 L1638 L1639 L1640 L1641 | L1642 L1643 L1644 L1645 L1646 L1647 | L1648 L1649 L1650 L1651 L1652 L1653 | L1654 L1655 L1656 L1657 L1658 L1659 | L1660 L1661 L1662 L1663 L1664 L1665 | L1666 L1667 L1668 L1669 L1670 L1671 | L1672 L1673 L1674 L1675 L1676 L1677 | L1678 L1679 L1680 L1681 L1682 L1683 | L1684 L1685 L1686 L1687 L1688 L1689 | L1690 L1691 L1692 L1693 L1694 L1695 | L1696 L1697 L1698 L1699 L1700 L1701 | L1702 L1703 L1704 L1705 L1706 L1707 | L1708 L1709 L1710 L1711 L1712 L1713 | L1714 L1715 L1716 L1717 L1718 L1719 | L1720 L1721 L1722 L1723 L1724 L1725 | L1726 L1727 L1728 L1729 L1730 L1731 | L1732 L1733 L1734 L1735 L1736 L1737 | L1738 L1739 L1740 L1741 L1742 L1743 | L1744 L1745 L1746 L1747 L1748 L1749 | L1750 L1751 L1752 L1753 L1754 L1755 | L1756 L1757 L1758 L1759 L1760 L1761 | L1762 L1763 L1764 L1765 L1766 L1767 | L1768 L1769 L1770 L1771 L1772 L1773 | L1774 L1775 L1776 L1777 L1778 L1779 | L1780 L1781 L1782 L1783 L1784 L1785 | L1786 L1787 L1788 L1789 L1790 L1791 | L1792 L1793 L1794 L1795 L1796 L1797 | L1798 L1799 L1800 L1801 L1802 L1803 | L1804 L1805 L1806 L1807 L1808 L1809 | L1810 L1811 L1812 L1813 L1814 L1815 | L1816 L1817 L1818 L1819 L1820 L1821 | L1822 L1823 L1824 L1825 L1826 L1827 | L1828 L1829 L1830 L1831 L1832 L1833 | L1834 L1835 L1836 L1837 L1838 L1839 | L1840 L1841 L1842 L1843 L1844 L1845 | L1846 L1847 L1848 L1849 L1850 L1851 | L1852 L1853 L1854 L1855 L1856 L1857 | L1858 L1859 L1860 L1861 L1862 L1863 | L1864 L1865 L1866 L1867 L1868 L1869 | L1870 L1871 L1872 L1873 L1874 L1875 | L1876 L1877 L1878 L1879 L1880 L1881 | L1882 L1883 L1884 L1885 L1886 L1887 | L1888 L1889 L1890 L1891 L1892 L1893 | L1894 L1895 L1896 L1897 L1898 L1899 | L1900 L1901 L1902 L1903 L1904 L1905 | L1906 L1907 L1908 L1909 L1910 L1911 | L1912 L1913 L1914 L1915 L1916 L1917 | L1918 L1919 L1920 L1921 L1922 L1923 | L1924 L1925 L1926 L1927 L1928 L1929 | L1930 L1931 L1932 L1933 L1934 L1935 | L1936 L1937 L1938 L1939 L1940 L1941 | L1942 L1943 L1944 L1945 L1946 L1947 | L1948 L1949 L1950 L1951 L1952 L1953 | L1954 L1955 L1956 L1957 L1958 L1959 | L1960 L1961 L1962 L1963 L1964 L1965 | L1966 L1967 L1968 L1969 L1970 L1971 | L1972 L1973 L1974 L1975 L1976 L1977 | L1978 L1979 L1980 L1981 L1982 L1983 | L1984 L1985 L1986 L1987 L1988 L1989 | L1990 L1991 L1992 L1993 L1994 L1995 | L1996 L1997 L1998 L1999 L2000 L2001 | L2002 L2003 L2004 L2005 L2006 L2007 | L2008 L2009 L2010 L2011 L2012 L2013 | L2014 L2015 L2016 L2017 L2018 L2019 | L2020 L2021 L2022 L2023 L2024 L2025 | L2026 L2027 L2028 L2029 L2030 L2031 | L2032 L2033 L2034 L2035 L2036 L2037 | L2038 L2039 L2040 L2041 L2042 L2043 | L2044 L2045 L2046 L2047 L2048 L2049 | L2050 L2051 L2052 L2053 L2054 L2055 | L2056 L2057 L2058 L2059 L2060 L2061 | L2062 L2063 L2064 L2065 L2066 L2067 | L2068 L2069 L2070 L2071 L2072 L2073 | L2074 L2075 L2076 L2077 L2078 L2079 | L2080 L2081 L2082 L2083 L2084 L2085 | L2086 L2087 L2088 L2089 L2090 L2091 | L2092 L2093 L2094 L2095 L2096 L2097 | L2098 L2099 L2100 L2101 L2102 L2103 | L2104 L2105 L2106 L2107 L2108 L2109 | L2110 L2111 L2112 L2113 L2114 L2115 | L2116 L2117 L2118 L2119 L2120 L2121 | L2122 L2123 L2124 L2125 L2126 L2127 | L2128 L2129 L2130 L2131 L2132 L2133 | L2134 L2135 L2136 L2137 L2138 L2139 | L2140 L2141 L2142 L2143 L2144 L2145 | L2146 L2147 L2148 L2149 L2150 L2151 | L2152 L2153 L2154 L2155 L2156 L2157 | L2158 L2159 L2160 L2161 L2162 L2163 | L2164 L2165 L2166 L2167 L2168 L2169 | L2170 L2171 L2172 L2173 L2174 L2175 | L2176 L2177 L2178 L2179 L2180 L2181 | L2182 L2183 L2184 L2185 L2186 L2187 | L2188 L2189 L2190 L2191 L2192 L2193 | L2194 L2195 L2196 L2197 L2198 L2199 | L2200 L2201 L2202 L2203 L2204 L2205 | L2206 L2207 L2208 L2209 L2210 L2211 | L2212 L2213 L2214 L2215 L2216 L2217 | L2218 L2219 L2220 L2221 L2222 L2223 | L2224 L2225 L2226 L2227 L2228 L2229 | L2230 L2231 L2232 L2233 L2234 L2235 | L2236 L2237 L2238 L2239 L2240 L2241 | L2242 L2243 L2244 L2245 L2246 L2247 | L2248 L2249 L2250 L2251 L2252 L2253 | L2254 L2255 L2256 L2257 L2258 L2259 | L2260 L2261 L2262 L2263 L2264 L2265 | L2266 L2267 L2268 L2269 L2270 L2271 | L2272 L2273 L2274 L2275 L2276 L2277 | L2278 L2279 L2280 L2281 L2282 L2283 | L2284 L2285 L2286 L2287 L2288 L2289 | L2290 L2291 L2292 L2293 L2294 L2295 | L2296 L2297 L2298 L2299 L2300 L2301 | L2302 L2303 L2304 L2305 L2306 L2307 | L2308 L2309 L2310 L2311 L2312 L2313 | L2314 L2315 L2316 L2317 L2318 L2319 | L2320 L2321 L2322 L2323 L2324 L2325 | L2326 L2327 L2328 L2329 L2330 L2331 | L2332 L2333 L2334 L2335 L2336 L2337 | L2338 L2339 L2340 L2341 L2342 L2343 | L2344 L2345 L2346 L2347 L2348 L2349 | L2350 L2351 L2352 L2353 L2354 L2355 | L2356 L2357 L2358 L2359 L2360 L2361 | L2362 L2363 L2364 L2365 L2366 L2367 | L2368 L2369 L2370 L2371 L2372 L2373 | L2374 L2375 L2376 L2377 L2378 L2379 | L2380 L2381 L2382 L2383 L2384 L2385 | L2386 L2387 L2388 L2389 L2390 L2391 | L2392 L2393 L2394 L2395 L2396 L2397 | L2398 L2399 L2400 L2401 L2402 L2403 | L2404 L2405 L2406 L2407 L2408 L2409 | L2410 L2411 L2412 L2413 L2414 L2415 | L2416 L2417 L2418 L2419 L2420 L2421 | L2422 L2423 L2424 L2425 L2426 L2427 | L2428 L2429 L2430 L2431 L2432 L2433 | L2434 L2435 L2436 L2437 L2438 L2439 | L2440 L2441 L2442 L2443 L2444 L2445 | L2446 L2447 L2448 L2449 L2450 L2451 | L2452 L2453 L2454 L2455 L2456 L2457 | L2458 L2459 L2460 L2461 L2462 L2463 | L2464 L2465 L2466 L2467 L2468 L2469 | L2470 L2471 L2472 L2473 L2474 L2475 | L2476 L2477 L2478 L2479 L2480 L2481 | L2482 L2483 L2484 L2485 L2486 L2487 | L2488 L2489 L2490 L2491 L2492 L2493 | L2494 L2495 L2496 L2497 L2498 L2499 | L2500 L2501 L2502 L2503 L2504 L2505 | L2506 L2507 L2508 L2509 L2510 L2511 | L2512 L2513 L2514 L2515 L2516 L2517 | L2518 L2519 L2520 L2521 L2522 L2523 | L2524 L2525 L2526 L2527 L2528 L2529 | L2530 L2531 L2532 L2533 L2534 L2535 | L2536 L2537 L2538 L2539 L2540 L2541 | L2542 L2543 L2544 L2545 L2546 L2547 | L2548 L2549 L2550 L2551 L2552 L2553 | L2554 L2555 L2556 L2557 L2558 L2559 | L2560 L2561 L2562 L2563 L2564 L2565 | L2566 L2567 L2568 L2569 L2570 L2571 | L2572 L2573 L2574 L2575 L2576 L2577 | L2578 L2579 L2580 L2581 L2582 L2583 | L2584 L2585 L2586 L2587 L2588 L2589 | L2590 L2591 L2592 L2593 L2594 L2595 | L2596 L2597 L2598 L2599 L2600 L2601 | L2602 L2603 L2604 L2605 L2606 L2607 | L2608 L2609 L2610 L2611 L2612 L2613 | L2614 L2615 L2616 L2617 L2618 L2619 | L2620 L2621 L2622 L2623 L2624 L2625 | L2626 L2627 L2628 L2629 L2630 L2631 | L2632 L2633 L2634 L2635 L2636 L2637 | L2638 L2639 L2640 L2641 L2642 L2643 | L2644 L2645 L2646 L2647 L2648 L2649 | L2650 L2651 L2652 L2653 L2654 L2655 | L2656 L2657 L2658 L2659 L2660 L2661 | L2662 L2663 L2664 L2665 L2666 L2667 | L2668 L2669 L2670 L2671 L2672 L2673 | L2674 L2675 L2676 L2677 L2678 L2679 | L2680 L2681 L2682 L2683 L2684 L2685 | L2686 L2687 L2688 L2689 L2690 L2691 | L2692 L2693 L2694 L2695 L2696 L2697 | L2698 L2699 L2700 L2701 L2702 L2703 | L2704 L2705 L2706 L2707 L2708 L2709 | L2710 L2711 L2712 L2713 L2714 L2715 | L2716 L2717 L2718 L2719 L2720 L2721 | L2722 L2723 L2724 L2725 L2726 L2727 | L2728 L2729 L2730 L2731 L2732 L2733 | L2734 L2735 L2736 L2737 L2738 L2739 | L2740 L2741 L2742 L2743 L2744 L2745 | L2746 L2747 L2748 L2749 L2750 L2751 | L2752 L2753 L2754 L2755 L2756 L2757 | L2758 L2759 L2760 L2761 L2762 L2763 | L2764 L2765 L2766 L2767 L2768 L2769 | L2770 L2771 L2772 L2773 L2774 L2775 | L2776 L2777 L2778 L2779 L2780 L2781 | L2782 L2783 L2784 L2785 L2786 L2787 | L2788 L2789 L2790 L2791 L2792 L2793 | L2794 L2795 L2796 L2797 L2798 L2799 | L2800 L2801 L2802 L2803 L2804 L2805 | L2806 L2807 L2808 L2809 L2810 L2811 | L2812 L2813 L2814 L2815 L2816 L2817 | L2818 L2819 L2820 L2821 L2822 L2823 | L2824 L2825 L2826 L2827 L2828 L2829 | L2830 L2831 L2832 L2833 L2834 L2835 | L2836 L2837 L2838 L2839 L2840 L2841 | L2842 L2843 L2844 L2845 L2846 L2847 | L2848 L2849 L2850 L2851 L2852 L2853 | L2854 L2855 L2856 L2857 L2858 L2859 | L2860 L2861 L2862 L2863 L2864 L2865 | L2866 L2867 L2868 L2869 L2870 L2871 | L2872 L2873 L2874 L2875 L2876 L2877 | L2878 L2879 L2880 L2881 L2882 L2883 | L2884 L2885 L2886 L2887 L2888 L2889 | L2890 L2891 L2892 L2893 L2894 L2895 | L2896 L2897 L2898 L2899 L2900 L2901 | L2902 L2903 L2904 L2905 L2906 L2907 | L2908 L2909 L2910 L2911 L2912 L2913 | L2914 L2915 L2916 L2917 L2918 L2919 | L2920 L2921 L2922 L2923 L2924 L2925 | L2926 L2927 L2928 L2929 L2930 L2931 | L2932 L2933 L2934 L2935 L2936 L2937 | L2938 L2939 L2940 L2941 L2942 L2943 | L2944 L2945 L2946 L2947 L2948 L2949 | L2950 L2951 L2952 L2953 L2954 L2955 | L2956 L2957 L2958 L2959 L2960 L2961 | L2962 L2963 L2964 L2965 L2966 L2967 | L2968 L2969 L2970 L2971 L2972 L2973 | L2974 L2975 L2976 L2977 L2978 L2979 | L2980 L2981 L2982 L2983 L2984 L2985 | L2986 L2987 L2988 L2989 L2990 L2991 | L2992 L2993 L2994 L2995 L2996 L2997 | L2998 L2999 L3000 L3001 L3002 L3003 | L3004 L3005 L3006 L3007 L3008 L3009 | L3010 L3011 L3012 L3013 L3014 L3015 | L3016 L3017 L3018 L3019 L3020 L3021 | L3022 L3023 L3024 L3025 L3026 L3027 | L3028 L3029 L3030 L3031 L3032 L3033 | L3034 L3035 L3036 L3037 L3038 L3039 | L3040 L3041 L3042 L3043 L3044 L3045 | L3046 L3047 L3048 L3049 L3050 L3051 | L3052 L3053 L3054 L3055 L3056 L3057 | L3058 L3059 L3060 L3061 L3062 L3063 | L3064 L3065 L3066 L3067 L3068 L3069 | L3070 L3071 L3072 L3073 L3074 L3075 | L3076 L3077 L3078 L3079 L3080 L3081